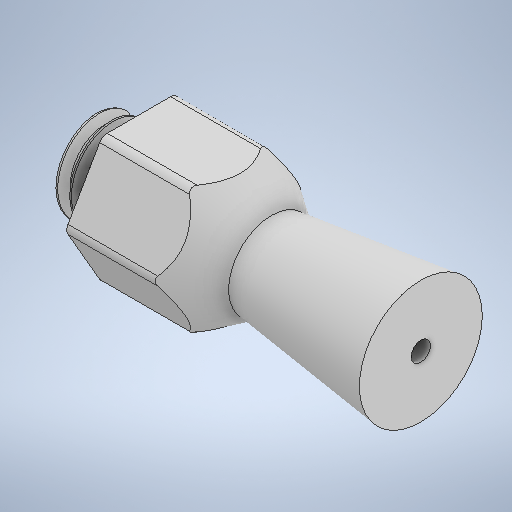
# Autodesk Inventor part: Part1
Saved by Autodesk Inventor 2025.2 (Build 292293000, 293)
## iProperties
Created: 2026-03-09
Part Number: Part1
Material: Generic
Document SubType Name: Modeling
Designer: Simon
Density: 1 g/cm^3
Appearance: Default
Author: Simon
Autodesk Inventor part; units mm, degrees
ref_plane "YZ Plane" through (0, 0, 0) normal (1, 0, 0) x (0, 1, 0)
ref_plane "XZ Plane" through (0, 0, 0) normal (0, 1, 0) x (-1, 0, 0)
ref_plane "XY Plane" through (0, 0, 0) normal (0, 0, 1) x (1, 0, 0)
sketch "Sketch1" plane through (0, 0, 0) normal (0, 0, 1) x (1, 0, 0)
  line L0 (0, 0) -> (0, 1.25)
  line L1 (0, 1.25) -> (50, 1.25)
  line L2 (0, 0) -> (0, 0.4819)
  line L3 (0, 0.4819) -> (50, 0.482)
  line L4 (0, 0) -> (0, 0.5574)
  line L5 (0, 0.5574) -> (50, 0.5574)
  line L6 (0, 0) -> (0, 2.5)
  line L7 (0, 2.5) -> (2.5, 2.5)
  line L8 (2.5, 2.5) -> (2.5, 1.25)
  line L9 (2.5, 1.25) -> (2.5, 4.25)
  line L10 (2.5, 1.25) -> (6.7109, 1.25) construction
  line L11 (2.5, 4.25) -> (7.5, 4.25)
  line L12 (7.5, 4.25) -> (7.5, 1.25)
  line L13 (7.5, 1.25) -> (10.1785, 0.482)
  line L14 (7.5, 1.25) -> (9.25, 1.25) construction
  line L15 (10.1785, 0.482) -> (18.8254, 0.5574)
  line L16 (10.1785, 0.482) -> (18.8257, 0.482) construction
  line L17 (18.8254, 0.5574) -> (18.8254, 3.5574)
  line L18 (10.1785, 0.482) -> (10.1785, 2.482)
  line L19 (10.1785, 2.482) -> (7.5, 4.25)
  line L20 (10.1785, 2.482) -> (18.8254, 3.5574)
  line L21 (0, 0) -> (50, 0)
  point P0 (2.5, 2.5)
  dimension "d0" = 1.25
  dimension "d1" = 50
  dimension "d2" = 0.4819
  dimension "d3" = 0.5574
  dimension "d4" = 2.5
  dimension "d5" = 2.5
  dimension "d6" = 3
  dimension "d8" = 5
  dimension "d9" = 16
  dimension "d10" = 0.5
  dimension "d12" = 3
  dimension "d13" = 2
  dimension "d14" = 50
  constraints: 44 end point, 8 perpendicular, 7 point on line, 5 horizontal, 2 vertical, 1 equal length
  measures "d0" distance of L0.start L0.end
  measures "d1" distance of L0.end L1.end
  measures "d2" distance of L0.start L2.end
  measures "d3" distance of L0.start L4.end
  measures "d4" distance of L0.start L6.end
  measures "d5" distance of L6.end L7.end
  measures "d6" distance of L8.end L9.end
  measures "d8" distance of L9.end L11.end
  measures "d9" angle of L13 L14
  measures "d10" angle of L16 L15
  measures "d12" distance of L15.end L17.end
  measures "d13" distance of L13.end L18.end
  measures "d14" distance of L0.start L21.end
revolve "Revolution1" add sketch "Sketch1" angle 360 about axis through (0, 0, 0) along (1, 0, 0) contours L18 L5 L15 | L13 L5 L18 | L6 L7 L8 L1 | L13 L1 L18 L5 | L5 L18 L1 L17 | L8 L9 L11 L12 L1 | L12 L19 L18 L1 | L1 L18 L20 L17
sketch "Sketch2" plane through (2.5, 0, 0) normal (-1, 0, 0) x (0, 0, 1)
  circle A0 centre (0, 0) radius 4.25 projected
  line L0 (2.125, 3.6806) -> (4.25, 0)
  line L1 (4.25, 0) -> (2.125, -3.6806)
  line L2 (2.125, -3.6806) -> (-2.125, -3.6806)
  line L3 (-2.125, -3.6806) -> (-4.25, 0)
  line L4 (-4.25, 0) -> (-2.125, 3.6806)
  line L5 (-2.125, 3.6806) -> (2.125, 3.6806)
  line L6 (-4.25, 0) -> (4.25, 0)
  circle A1 centre (0, 0) radius 1.25
  point P0 (-4.25, 0)
  point P1 (-4.25, 0)
  point P2 (2.125, -3.6806)
  point P3 (2.125, -3.6806)
  constraints: 14 end point, 3 point on circle, 2 coincident, 1 centre point, 1 horizontal, 1 parallel, 13 other
extrude "Extrusion1" cut sketch "Sketch2" against normal through all contours L0 A0 | A0 L1 | L5 A0 | A0 L2 | L4 A0 | A0 L3
fillet "Fillet1" radius 0.5 6 edges at (5, 3.6806, -2.125) (5, 3.6806, 2.125) (5, 0, 4.25) (5, -3.6806, 2.125) (5, -3.6806, -2.125) (5, 0, -4.25)
sketch "Sketch3" plane through (0, 0, 0) normal (-1, 0, 0) x (0, 0, 1)
  circle A0 centre (0, 0) radius 2.5 projected
  point P0 (0, 2.5)
  constraints: 1 vertical alignment, 1 other
sketch "Sketch4" plane through (0, 0, 0) normal (0, 0, 1) x (1, 0, 0)
  line L0 (-0.35, 1.8938) -> (0.45, 1.8938)
  line L1 (-0.35, 1.8938) -> (0.05, 2.5866)
  line L2 (-0.35, 1.8938) -> (0.45, 1.8938) construction
  line L3 (0.05, 2.5866) -> (0.45, 1.8938)
  line L4 (0.05, 2.5866) -> (0.85, 2.5866) construction
  line L5 (0.05, 2.5866) -> (0.05, 1.8938)
  line L6 (0.05, 1.8938) -> (0.05, 2.0671)
  line L7 (0.05, 2.0671) -> (0.45, 2.0671)
  line L8 (0.45, 2.0671) -> (-0.35, 2.0671)
  line L9 (0.05, 2.5866) -> (0.05, 2.5)
  line L10 (0.05, 2.5) -> (0.45, 2.5)
  line L11 (0.45, 2.5) -> (-0.35, 2.5)
  line L12 (-0.35, 1.8938) -> (-1.15, 1.8938)
  line L13 (0.05, 2.5866) -> (-0.75, 2.5866)
  line L14 (-0.75, 2.5866) -> (-1.15, 1.8938)
  line L15 (-0.35, 1.8938) -> (-0.75, 2.5866)
  line L16 (-0.35, 2.0671) -> (-1.15, 2.0671)
  line L17 (-0.35, 2.5) -> (-0.8, 2.5)
  line L18 (-0.75, 2.5866) -> (-0.75, 1.8938)
  line L19 (-0.35, 1.8938) -> (-0.35, 1.9938)
  circle A0 centre (-0.35, 2.0938) radius 0.1
  line L20 (-0.4077, 1.9938) -> (-0.2923, 1.9938)
  line L21 (0, -2.5) -> (0, 2.5) projected
  line L22 (-0.4366, 2.0438) -> (-0.2634, 2.0438)
  line L23 (-0.2634, 2.0438) -> (0, 2.5)
  line L24 (-0.7, 2.5) -> (0, 2.5)
  line L25 (-0.7, 2.5) -> (-0.4366, 2.0438)
  circle A1 centre (-0.35, 2.0938) radius 0.1
  point P0 (0, 0)
  dimension "d19" = 0.8
  dimension "d20" = 60
  dimension "d21" = 60
  dimension "d22" = 0.1732
  dimension "d23" = 0.0866
  dimension "d24" = 0.8
  dimension "d25" = 0.1
  dimension "d26" = 0.8
  constraints: 50 end point, 12 point on line, 7 horizontal, 4 tangent, 3 collinear, 3 midpoint, 2 equal length, 2 perpendicular, 2 point on circle, 1 centre point, 1 coincident, 1 parallel, 1 vertical, 3 other
  measures "d19" distance of L0.start L0.end
  measures "d20" angle of L2 L1
  measures "d21" angle of L3 L4
  measures "d22" distance of L5.end L6.end
  measures "d23" distance of L1.end L9.end
  measures "d24" distance of L0.start L12.end
  measures "d25" distance of L0.start L19.end
  measures "d26" distance between parallel lines of L5 L18
coil "Coil1" sketch "Sketch4" operation cut axis through (-10, 0, 0) along (1, 0, 0) pitch 0.8 turns 4 hand right contours A0 L22 | A0 L15 L17 L11 L1 | L1 L22 L15 L16 L8 | L8 L16 A0 | L11 L17 L15 L13 L1
extrude "Extrusion4" add sketch "Sketch2" against normal blind 5 contours L6 A1 L4 L5 L0 | L1 L2 L3 L6 A1
fillet "Fillet3" radius 0.5 6 edges at (5, 3.6806, -2.125) (5, 3.6806, 2.125) (5, 0, 4.25) (5, -3.6806, 2.125) (5, -3.6806, -2.125) (5, 0, -4.25)
body "Solid1"
